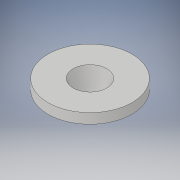
# Autodesk Inventor part: clamp_cup
Saved by Autodesk Inventor 2019.3 (Build 233278000, 278)
## iProperties
Created: 2019-04-14
Part Number: clamp_cup
Material: Generic
Document SubType Name: Modeling
Designer: peter
Density: 1 g/cm^3
Appearance: Default
Author: peter
Autodesk Inventor part; units mm, degrees
ref_plane "YZ Plane" through (0, 0, 0) normal (1, 0, 0) x (0, 1, 0)
ref_plane "XY Plane" through (0, 0, 0) normal (0, 0, 1) x (1, 0, 0)
sketch "Sketch1" plane through (0, 0, 0) normal (0, 1, 0) x (-1, 0, 0)
  circle A0 centre (0, 0) radius 12.5
  circle A1 centre (0, 0) radius 5
  dimension "d0" = 25
  dimension "d1" = 10
  constraints: 2 centre point, 2 coincident
  measures "d0" diameter of A0
  measures "d1" diameter of A1
ref_plane "Work Plane1" through (0, -6, 0) normal (0, 1, 0) x (-1, 0, 0)
sketch "Sketch2" plane through (0, -6, 0) normal (0, 1, 0) x (-1, 0, 0)
  circle A0 centre (0, 0) radius 3
  circle A1 centre (0, 0) radius 5
  dimension "d3" = 6
  dimension "d4" = 10
  constraints: 2 centre point, 2 coincident
  measures "d3" diameter of A0
  measures "d4" diameter of A1
sketch "Sketch3" plane through (0, 0, 0) normal (1, 0, 0) x (0, 1, 0)
  line L0 (-6, -5) -> (-6, 5) projected
  line L1 (0, -12.5) -> (0, 12.5) projected
  line L2 (0, 12.5) -> (-3, 12.5)
  line L3 (0, 12.5) -> (3, 12.5) construction
  arc A0 (-6, 5) -> (-3, 12.5) centre (-13.4109, 12.3144) ccw
  line L4 (0, -5) -> (0, 5) projected
  line L5 (-6, -3) -> (-6, 3) projected
  line L6 (0, 5) -> (-6, 3)
  line L7 (-16.6931, 0) -> (6.2822, 0) projected
  point P0 (0, 0)
  dimension "d5" = 3
  dimension "d6" = 180
  constraints: 6 end point, 2 horizontal, 2 point on circle, 1 centre point, 1 collinear
  measures "d5" distance of L1.end L2.end
  measures "d6" angle of L2 L3
revolve "Revolution1" add sketch "Sketch3" angle 360 about axis through (0, -10, 0) along (0, 1, 0) contours L0 A0 L2 L1 L6
body "Solid1"
